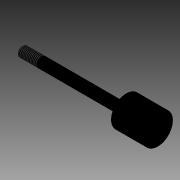
# Autodesk Inventor part: C-040.5-RP0000_rod
Saved by Autodesk Inventor 2014 SP2 (Build 180246200, 246)
## iProperties
Created: 2019-01-25
Part Number: C-040.5-RP0000_rod
Material: Generic
Catalog Web Link: www.cadenas.de
Description: Standard Air Cylinder_rod-Original Line - Standard Air Cylinders
Vendor: BIMBA
Document SubType Name: Modeling
Designer: psadmin
Manufacturer: BIMBA
Mass: 7.88731 g
Surface Area: 31.0529 cm^2
Volume: 7.88731 cm^3
Density: 1 g/cm^3
Appearance: PSOLRGB-0-0-0
Category: PARTsolutions
Company: BIMBA
Title: C-040.5-RP0000_rod
Author: Cadenas PARTsolutions
Comments: Original Line - Standard Air Cylinders
PSOL_IDENT_0: {$CADENAS_DATA\23d-libs\bimba\bimba\bimba_imperial\bimba_full_line\original_line_cylinders\standard_
PSOL_IDENT_1: air_cylinders\rod.prj},329 {VTYP=3D},{NB=C-040.5-RP0000_rod},{LINA=C-040.5-RP0000_rod},{NN=Standard
PSOL_IDENT_2: Air Cylinder_rod},{DATE=21.03.2018 14:31:21},{GEOMDATE=09.11.2017 13:09:15},{VERSION=},{LINEID=50},{
PSOL_IDENT_3: WBVAR=STROKE,ACTING,MNT,DER,NR,BM,CO,M,EE,EEL,K,Q,Y,F,G,T,B,H,SER,SR,NT,W,E,HL,ST,STP,PRC,PB,COLOR1,
PSOL_IDENT_4: FCD,RCD,BCD},{WBNUMERIC=STROKE,EEL,COLOR1,FCD,RCD,BCD}  {NB=C-040.5-RP0000_rod},{LINA=C-040.5-RP0000
PSOL_IDENT_5: _rod},{KT=DUMMY},{PN=C-040.5-RP000},{DASH=-},{BORE=0.75000000},{BOREPN=04},{STROKE=0.500},{STROKEALG=
PSOL_IDENT_6: [0.001:50/0.001]},{STROKE1=0.500},{ACTING=R},{ACTINGALG= '' , 'Single Acting' , 'R' , 'Reverse Singl
PSOL_IDENT_7: e Acting' , 'D' , 'Double Acting' },{ACTINGPN=R},{MNT=P},{MNTALG= '' , 'Front Nose Mounting' , 'P' ,
PSOL_IDENT_8: 'Rear Pivot Mounting' , 'BF' , 'Front Block Mounting' , 'BR' , 'Rear Block Mounting for Vertical Po
PSOL_IDENT_9: sitioning' , 'A' , 'Nose Mounting with Adjustable Stroke' },{TYPE=C-},{MNTPN=P},{DER=},{DERALG= '' ,
PSOL_IDENT_10: 'N/A' },{NR=},{NRALG= '' , 'N/A' },{NRPN=},{BM=},{BMALG= '' , 'N/A' },{BMPN=},{CO=},{COALG= '' , 'N
PSOL_IDENT_11: /A' },{M=},{MALG= '', 'Without Magnet', 'M', 'With Magnet' },{EE=},{EEL=0},{EEMAX=12},{EEALG= '', 'W
PSOL_IDENT_12: ithout Extra Extension', 'EE', 'With Extra Extension' },{EELALG=0},{EEPN=},{EEPN1=0.000},{K=},{KALG=
PSOL_IDENT_13: '', 'Standard' , 'K' , 'Ports Rotated 90deg' },{KPN=},{Q=},{QALG= '' , 'Without Side Ported Rear He
PSOL_IDENT_14: ad' , 'Q' , 'With Side Ported Rear Head' },{QPN=},{Y=},{YALG= '' , 'Without Pivot Bushing' , 'Y' , '
PSOL_IDENT_15: With Pivot Bushing' },{YPN=},{F=},{FALG= '', 'Standard', 'F', 'Molycoated Body' },{FPN=},{G=},{GPN=}
PSOL_IDENT_16: ,{T=},{TALG= '' , 'Standard' , 'N' , 'Low Temperature' , 'V' , 'High Temperature' },{NPN=},{VPN=},{B=
PSOL_IDENT_17: },{BALG= '', 'Without Bumper' , 'B' , 'With Bumper' },{BPN=},{H=},{HALG= '', 'Standard', 'H', 'With
PSOL_IDENT_18: Heavy Springs' },{HPN=},{SER=},{SERALG= '' , 'N/A' },{SR=C},{SRALG= 'C' , 'Carbon Steel Rod' , 'SR'
PSOL_IDENT_19: , '303 Stainless Steel Rod' , '' , '303 Stainless Steel Rod1' },{SRPN=C},{SRCON=1},{NT=},{NTPN=},{W=
PSOL_IDENT_20: },{WALG= '' , 'Without Wiper' , 'W' , 'With Wiper' },{WPN=},{E=},{EALG= '' , 'Without Special Lube a
PSOL_IDENT_21: nd Seals' , 'E' , 'With Special Lube and Seals' },{EPN=},{HL=},{HLALG= '' , 'N/A' },{ST=},{STALG= ''
PSOL_IDENT_22: , 'Without Switch Track' , 'T' , 'With Switch Track' },{STP=},{STPALG= '' , 'N/A' },{STPN=},{PRC=},
PSOL_IDENT_23: {PRCALG= '' , 'Without Piston Rod Clevis' , 'D-166-1' , 'With Piston Rod Clevis' },{PRCPN=},{PB=},{P
PSOL_IDENT_24: BALG= '' , 'Without Pivot Bracket' , 'D-167' , 'With Pivot Bracket' },{PBPN=},{TLEN=1.7595},{TEXT=0.
PSOL_IDENT_25: 133333},{SPACE=0.07619},{FRAC=4.1300},{RGCON=},{RGDACCON=R},{RHCON=P},{RHCONON=1},{RHACCON=R},{FNUTC
PSOL_IDENT_26: ON=0},{RNUTCON=0},{FNUTPN=},{RNUTPN=},{FNUTTRANS=0.0000},{RNUTTRANS=0.0000},{VHOLECON=3},{A1=1.5940}
PSOL_IDENT_27: ,{A1N=0.8750},{A1P=1.5940},{A1B=1.5940},{A4=0.2525},{A4N=0.3130},{A4P=0.2525},{A5=0.0300},{A1H=0.278
PSOL_IDENT_28: 5},{A1NH=0.5310},{A1PH=1.5940},{A1BH=1.0940},{A1SH=1.2190},{A2H=0.1560},{A2NH=0.2190},{LENGTH=2.4400
PSOL_IDENT_29: },{LENGTH1=2.4400},{LENGTH2=3.8100},{MUL=1.3450},{MUL11=1.3450},{MUL22=1.3450},{MUL33=0.8450},{MUL2=
PSOL_IDENT_30: 2.6900},{MUL211=2.6900},{MUL222=2.6900},{MUL233=1.6900},{SSS=0.5000},{RGLEN=1.3715},{RHLEN=0.4990},{
PSOL_IDENT_31: SSS1=1.0000},{A13=1.3120},{THDLEN1=0.5000},{THD1=0.2500},{TAB=UNF},{THDLEN=0.5000},{THD=0.2500},{OD=
PSOL_IDENT_32: 0.7615},{RODL=3.3800},{PL=0.7860},{RODDIA=0.2500},{HEX=0.2500},{RODTRANS=0.5000},{G1=0.1250},{ON=1},
PSOL_IDENT_33: {G5=0.6250},{DERLEN=2.5940},{THOLE=0.0000},{WF=0.2200},{BADD=0.0000},{MADD=0.0000},{NVADD=0.000},{JR
PSOL_IDENT_34: ADD=0.00000},{COLOR=0.00,0.00,0.00,0.00},{GROOVE=1},{HOL=0},{D7=0.2520},{H1=1.1175},{D1=0.8625},{D1R
PSOL_IDENT_35: H=0.8050},{D1P=0.8325},{D1B=0.8625},{D1N=0.8050},{D1NRH=0.8050},{D1BRH=0.8325},{D1PRH=0.8625},{BOZO=
PSOL_IDENT_36: 1},{HADD=0.000},{COLOR1=0},{DEFL=0.0000},{HEXL=0.0000},{SSADD=0.0000},{WFL=0.0000},{MOVE=0.0000},{PR
PSOL_IDENT_37: CL2=0.50000},{PRCB=0.16000},{PRCTRANS=0.16000},{FCD=0},{RCD=0},{BCD=0}
NN: Standard Air Cylinder_rod
NT: Standard
NB: C-040.5-RP0000_rod
NBSYN: $PN.$COLOR1._rod
LINA: C-040.5-RP0000_rod
PN: C-040.5-RP000
BORE: 0.75
BOREPN: 04
STROKE: 0.5
ACTING: Reverse Single Acting
MNT: Rear Pivot Mounting
DER: N/A
NR: N/A
BM: N/A
CO: N/A
M: Without Magnet
EE: Without Extra Extension
EEL: 0
K: Standard
Q: Without Side Ported Rear Head
Y: Without Pivot Bushing
F: Standard
G: Without Magnalube Lubrication
T: Standard
B: Without Bumper
H: Standard
SER: N/A
SR: Carbon Steel Rod
W: Without Wiper
E: Without Special Lube and Seals
HL: N/A
ST: Without Switch Track
STP: N/A
PRC: Without Piston Rod Clevis
PB: Without Pivot Bracket
A1N: 0.875
A1P: 1.594
A1B: 1.594
A4N: 0.313
A4P: 0.2525
A5: 0.03
A1NH: 0.531
A1PH: 1.594
A1BH: 1.094
A1SH: 1.219
A2NH: 0.219
A13: 1.312
THDLEN1: 0.5
THD1: 0.25
TAB: UNF
OD: 0.7615
RODDIA: 0.25
HEX: 0.25
G1: 0.125
G5: 0.625
THOLE: 0
WF: 0.22
GROOVE: 1
D7: 0.252
D1P: 0.8325
D1B: 0.8625
D1N: 0.805
D1NRH: 0.805
D1BRH: 0.8325
D1PRH: 0.8625
COLOR1: 0
FCD: 0
RCD: 0
BCD: 0
SUPPLIER: BIMBA
ARTICLENO: C-040.5-RP0000_rod
BOMINFO: C-040.5-RP0000_rod
CREATOR: CADENAS GmbH
Autodesk Inventor part; units mm, degrees
sketch "Sketch_1" plane through (0, 0, 0) normal (0, 0, 1) x (1, 0, 0)
  line L0 (73.152, 0) -> (0, 0)
  line L1 (0, 0) -> (0, 3.175)
  line L2 (0, 3.175) -> (53.1876, 3.175)
  line L3 (53.1876, 3.175) -> (53.1876, 9.6203)
  line L4 (53.1876, 9.6203) -> (73.152, 9.6203)
  line L5 (73.152, 9.6203) -> (73.152, 0)
  line L6 (73.152, 0) -> (0, 0)
  constraints: 14 end point
revolve "Revolution1" add sketch "Sketch_1" angle 360 about axis through (73.152, 0, 0) along (1, 0, 0)
sketch "Sketch_3" plane through (0, 0, 0) normal (0, 0, 1) x (1, 0, 0)
  line L0 (0, 0) -> (-12.7, 0)
  line L1 (-12.7, 0) -> (-12.7, 2.634)
  line L2 (-12.7, 2.634) -> (-12.159, 3.175)
  line L3 (-12.159, 3.175) -> (0, 3.175)
  line L4 (0, 3.175) -> (0, 0)
  line L5 (0, 0) -> (-12.7, 0)
  constraints: 12 end point
revolve "Revolution2" add sketch "Sketch_3" angle 360 about axis through (0, 0, 0) along (1, 0, 0)
thread "Thread1" size "1/4-28 UNF" class "2A" standard "ANSI Unified Screw Threads" length 12.159
sketch "Sketch_30" plane through (0, 0, 0) normal (0, 0, 1) x (1, 0, 0)
  line L0 (0, 0) -> (-0.254, 0)
  line L1 (-0.254, 2.921) -> (0, 2.921)
  line L2 (0, 2.921) -> (0, 3.429)
  line L3 (0, 3.429) -> (-0.254, 3.429)
  line L4 (-0.254, 3.429) -> (-0.254, 2.921)
  constraints: 10 end point
revolve "Revolution3" cut sketch "Sketch_30" angle 360 about axis through (0, 0, 0) along (1, 0, 0)
ref_plane "dia1_XY" through (0, 3.175, 0) normal (1, 0, 0) x (0, 0, -1)
ref_plane "dia1_YZ" through (0, 3.175, 0) normal (0, 0, -1) x (0, 1, 0)
ref_plane "dia1_ZX" through (0, 3.175, 0) normal (0, 1, 0) x (1, 0, 0)
ref_plane "dia12_XY" through (0, 0, 10.9537) normal (1, 0, 0) x (0, 0, -1)
ref_plane "dia12_YZ" through (0, 0, 10.9537) normal (0, 0, -1) x (0, 1, 0)
ref_plane "dia12_ZX" through (0, 0, 10.9537) normal (0, 1, 0) x (1, 0, 0)
ref_plane "dia1r_XY" through (0, 0, 10.2235) normal (1, 0, 0) x (0, 0, -1)
ref_plane "dia1r_YZ" through (0, 0, 10.2235) normal (0, 0, -1) x (0, 1, 0)
ref_plane "dia1r_ZX" through (0, 0, 10.2235) normal (0, 1, 0) x (1, 0, 0)
ref_plane "dia2_XY" through (0, -3.175, 0) normal (1, 0, 0) x (0, 0, -1)
ref_plane "dia2_YZ" through (0, -3.175, 0) normal (0, 0, -1) x (0, 1, 0)
ref_plane "dia2_ZX" through (0, -3.175, 0) normal (0, 1, 0) x (1, 0, 0)
ref_plane "dia22_XY" through (0, 0, -10.9537) normal (1, 0, 0) x (0, 0, -1)
ref_plane "dia22_YZ" through (0, 0, -10.9537) normal (0, 0, -1) x (0, 1, 0)
ref_plane "dia22_ZX" through (0, 0, -10.9537) normal (0, 1, 0) x (1, 0, 0)
ref_plane "dia2r_XY" through (0, 0, -10.2235) normal (1, 0, 0) x (0, 0, -1)
ref_plane "dia2r_YZ" through (0, 0, -10.2235) normal (0, 0, -1) x (0, 1, 0)
ref_plane "dia2r_ZX" through (0, 0, -10.2235) normal (0, 1, 0) x (1, 0, 0)
ref_plane "rl1_XY" through (-12.7, 0, 0) normal (1, 0, 0) x (0, 0, -1)
ref_plane "rl1_YZ" through (-12.7, 0, 0) normal (0, 0, -1) x (0, 1, 0)
ref_plane "rl1_ZX" through (-12.7, 0, 0) normal (0, 1, 0) x (1, 0, 0)
ref_plane "rl2_XY" through (0, 0, 0) normal (1, 0, 0) x (0, 0, -1)
ref_plane "rl2_YZ" through (0, 0, 0) normal (0, 0, -1) x (0, 1, 0)
ref_plane "rl2_ZX" through (0, 0, 0) normal (0, 1, 0) x (1, 0, 0)
ref_plane "rod_cp_XY" through (0, 0, 0) normal (1, 0, 0) x (0, 0, -1)
ref_plane "rod_cp_YZ" through (0, 0, 0) normal (0, 0, -1) x (0, 1, 0)
ref_plane "rod_cp_ZX" through (0, 0, 0) normal (0, 1, 0) x (1, 0, 0)
ref_plane "stroke1_XY" through (0, 0, 0) normal (1, 0, 0) x (0, 0, -1)
ref_plane "stroke1_YZ" through (0, 0, 0) normal (0, 0, -1) x (0, 1, 0)
ref_plane "stroke1_ZX" through (0, 0, 0) normal (0, 1, 0) x (1, 0, 0)
ref_plane "thd1_XY" through (-12.7, 3.175, 0) normal (1, 0, 0) x (0, 0, -1)
ref_plane "thd1_YZ" through (-12.7, 3.175, 0) normal (0, 0, -1) x (0, 1, 0)
ref_plane "thd1_ZX" through (-12.7, 3.175, 0) normal (0, 1, 0) x (1, 0, 0)
ref_plane "thd2_XY" through (-12.7, -3.175, 0) normal (1, 0, 0) x (0, 0, -1)
ref_plane "thd2_YZ" through (-12.7, -3.175, 0) normal (0, 0, -1) x (0, 1, 0)
ref_plane "thd2_ZX" through (-12.7, -3.175, 0) normal (0, 1, 0) x (1, 0, 0)
ref_plane "to_rod_clevis_XY" through (-16.764, 0, 0) normal (1, 0, 0) x (0, 0, -1)
ref_plane "to_rod_clevis_YZ" through (-16.764, 0, 0) normal (0, 0, -1) x (0, 1, 0)
ref_plane "to_rod_clevis_ZX" through (-16.764, 0, 0) normal (0, 1, 0) x (1, 0, 0)
body "Solid1"
